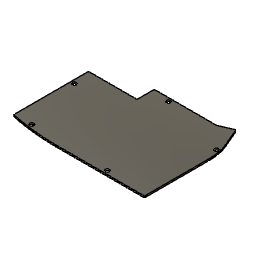
bottom plate lily58 v7 (Autodesk Fusion 360 design; units mm, degrees)
Autodesk Fusion 360 part; units mm, degrees
note: some values were not read from the file. Set by a fixed rule: which sketch regions a step uses.
sketch "bottom plate template" plane through (0, 0, 0) normal (0, 0, 1) x (1, 0, 0)
  line L0 (-42.4011, 43.5515) -> (-42.2701, 43.5244)
  line L1 (-42.5272, 43.5961) -> (-42.4011, 43.5515)
  line L2 (-42.2701, 43.5244) -> (-42.1367, 43.5153)
  line L3 (-55.1253, 50.5809) -> (-54.9545, 50.5783)
  line L4 (-64.5273, 28.4738) -> (-65.371, 25.3295)
  line L5 (-66.7867, 15.6775) -> (-66.8817, 12.4194)
  line L6 (-55.5934, 50.1095) -> (-62.3002, 34.5844)
  line L7 (-41.9037, 44.9516) -> (-41.9486, 44.9547)
  line L8 (-41.9486, 44.9547) -> (-42.014, 44.9682)
  line L9 (-42.1092, 45.0018) -> (-54.8288, 50.4967)
  line L10 (-63.502, 31.5638) -> (-64.5273, 28.4738)
  line L11 (-54.9545, 50.5783) -> (-55.1711, 50.5238)
  line L12 (-65.371, 25.3295) -> (-66.0302, 22.1414)
  line L13 (-55.1711, 50.5238) -> (-55.3484, 50.4249)
  line L14 (-55.4828, 50.2945) -> (-55.5934, 50.1095)
  line L15 (-66.0302, 22.1414) -> (-66.5026, 18.9204)
  line L16 (19.5634, 28.0336) -> (19.4331, 28.1336)
  line L17 (19.2505, 44.285) -> (19.2271, 44.463)
  line L18 (19.2711, 28.414) -> (19.2505, 28.5705)
  line L19 (19.2271, 44.463) -> (19.1628, 44.6182)
  line L20 (-66.8598, -50.3716) -> (-66.7963, -50.5251)
  line L21 (19.2505, 28.5705) -> (19.2505, 44.285)
  line L22 (66.8473, 27.4924) -> (66.7857, 27.641)
  line L23 (-62.3002, 34.5844) -> (-63.502, 31.5638)
  line L24 (19.4331, 28.1336) -> (19.3335, 28.2635)
  line L25 (25.9383, -50.737) -> (32.7303, -50.4296)
  line L26 (66.8528, -45.3702) -> (66.8694, -45.2242)
  line L27 (66.8694, -45.2242) -> (66.8694, 27.3244)
  line L28 (-42.014, 44.9682) -> (-42.1092, 45.0018)
  line L29 (-54.8288, 50.4967) -> (-55.1253, 50.5809)
  line L30 (39.5099, -49.9176) -> (46.2711, -49.2014)
  line L31 (-66.8817, 12.4194) -> (-66.8817, -50.2057)
  line L32 (-66.5666, -50.755) -> (-66.4167, -50.8171)
  line L33 (66.2436, 27.9503) -> (19.8699, 27.9503)
  line L34 (19.1392, -50.8395) -> (25.9383, -50.737)
  line L35 (19.1628, 44.6182) -> (19.0586, 44.754)
  line L36 (-66.6961, -50.6556) -> (-66.5666, -50.755)
  line L37 (-55.3484, 50.4249) -> (-55.4828, 50.2945)
  line L38 (66.8694, 27.3244) -> (66.8473, 27.4924)
  line L39 (19.0586, 44.754) -> (18.9193, 44.8609)
  line L40 (66.5601, 27.8666) -> (66.4114, 27.9282)
  line L41 (18.5904, 44.9516) -> (-41.9037, 44.9516)
  line L42 (53.0076, -48.2817) -> (59.7132, -47.1593)
  line L43 (19.8699, 27.9503) -> (19.7156, 27.9706)
  line L44 (18.7515, 44.9304) -> (18.5904, 44.9516)
  line L45 (-66.8817, -50.2057) -> (-66.8598, -50.3716)
  line L46 (18.9193, 44.8609) -> (18.7515, 44.9304)
  line L47 (-66.246, -50.8395) -> (19.1392, -50.8395)
  line L48 (19.7156, 27.9706) -> (19.5634, 28.0336)
  line L49 (-66.7963, -50.5251) -> (-66.6961, -50.6556)
  line L50 (66.7857, 27.641) -> (66.6878, 27.7686)
  line L51 (66.4114, 27.9282) -> (66.2436, 27.9503)
  line L52 (19.3335, 28.2635) -> (19.2711, 28.414)
  line L53 (66.8063, -45.5016) -> (66.8528, -45.3702)
  line L54 (66.632, -45.7171) -> (66.7315, -45.6193)
  line L55 (59.7132, -47.1593) -> (66.3751, -45.8367)
  line L56 (46.2711, -49.2014) -> (53.0076, -48.2817)
  line L57 (66.5131, -45.7902) -> (66.632, -45.7171)
  line L58 (66.7315, -45.6193) -> (66.8063, -45.5016)
  line L59 (66.6878, 27.7686) -> (66.5601, 27.8666)
  line L60 (66.3751, -45.8367) -> (66.5131, -45.7902)
  line L61 (32.7303, -50.4296) -> (39.5099, -49.9176)
  line L62 (-66.5026, 18.9204) -> (-66.7867, 15.6775)
  line L63 (-66.4167, -50.8171) -> (-66.246, -50.8395)
  circle A0 centre (1.8529, 41.4534) radius 1.5
  circle A1 centre (63.2875, 10.5583) radius 1.5
  circle A2 centre (49.4779, -45.0902) radius 1.5
  circle A3 centre (-26.7221, -47.1013) radius 1.5
  circle A4 centre (-62.68, 23.9748) radius 1.5
  circle A5 centre (-62.68, 23.9748) radius 2
  circle A6 centre (1.8529, 41.4534) radius 2
  circle A7 centre (49.4779, -45.0902) radius 2
  circle A8 centre (-26.7221, -47.1013) radius 2
  circle A9 centre (63.2875, 10.5583) radius 2
  line L64 (-41.9622, 44.8554) -> (-42.041, 44.8716)
  line L65 (-42.041, 44.8716) -> (-42.1457, 44.9087)
  line L66 (-42.1457, 44.9087) -> (-54.8625, 50.4023)
  line L67 (-54.8625, 50.4023) -> (-55.0418, 50.4532)
  line L68 (-55.0418, 50.4532) -> (-55.1339, 50.43)
  line L69 (-55.1339, 50.43) -> (-55.2883, 50.344)
  line L70 (-55.2883, 50.344) -> (-55.4037, 50.2319)
  line L71 (-55.4037, 50.2319) -> (-55.5042, 50.0638)
  line L72 (-55.5042, 50.0638) -> (-62.2079, 34.5461)
  line L73 (-62.2079, 34.5461) -> (-63.408, 31.5295)
  line L74 (-63.408, 31.5295) -> (-64.4315, 28.4451)
  line L75 (-64.4315, 28.4451) -> (-65.2737, 25.3064)
  line L76 (-65.2737, 25.3064) -> (-65.9317, 22.124)
  line L77 (-65.9317, 22.124) -> (-66.4033, 18.9088)
  line L78 (-66.4033, 18.9088) -> (-66.6869, 15.6717)
  line L79 (-66.6869, 15.6717) -> (-66.7817, 12.4179)
  line L80 (-66.7817, 12.4179) -> (-66.7817, -50.1991)
  line L81 (-66.7817, -50.1991) -> (-66.7624, -50.3455)
  line L82 (-66.7624, -50.3455) -> (-66.7089, -50.4747)
  line L83 (-66.7089, -50.4747) -> (-66.6248, -50.5843)
  line L84 (-66.6248, -50.5843) -> (-66.5162, -50.6676)
  line L85 (-66.5162, -50.6676) -> (-66.3905, -50.7197)
  line L86 (-66.3905, -50.7197) -> (-66.2395, -50.7395)
  line L87 (-66.2395, -50.7395) -> (19.1385, -50.7395)
  line L88 (19.1385, -50.7395) -> (25.9352, -50.6371)
  line L89 (25.9352, -50.6371) -> (32.7243, -50.3298)
  line L90 (32.7243, -50.3298) -> (39.5009, -49.818)
  line L91 (39.5009, -49.818) -> (46.2591, -49.1021)
  line L92 (46.2591, -49.1021) -> (52.9925, -48.1828)
  line L93 (52.9925, -48.1828) -> (59.6952, -47.0609)
  line L94 (59.6952, -47.0609) -> (66.3493, -45.7398)
  line L95 (66.3493, -45.7398) -> (66.4705, -45.6991)
  line L96 (66.4705, -45.6991) -> (66.57, -45.6379)
  line L97 (66.57, -45.6379) -> (66.6532, -45.556)
  line L98 (66.6532, -45.556) -> (66.7158, -45.4576)
  line L99 (66.7158, -45.4576) -> (66.7547, -45.3476)
  line L100 (66.7547, -45.3476) -> (66.7694, -45.2185)
  line L101 (66.7694, -45.2185) -> (66.7694, 27.3178)
  line L102 (66.7694, 27.3178) -> (66.7498, 27.4663)
  line L103 (66.7498, 27.4663) -> (66.6984, 27.5906)
  line L104 (66.6984, 27.5906) -> (66.6165, 27.6973)
  line L105 (66.6165, 27.6973) -> (66.5097, 27.7792)
  line L106 (66.5097, 27.7792) -> (66.3853, 27.8308)
  line L107 (66.3853, 27.8308) -> (66.2371, 27.8503)
  line L108 (66.2371, 27.8503) -> (19.8634, 27.8503)
  line L109 (19.8634, 27.8503) -> (19.6895, 27.8732)
  line L110 (19.6895, 27.8732) -> (19.513, 27.9463)
  line L111 (19.513, 27.9463) -> (19.3618, 28.0623)
  line L112 (19.3618, 28.0623) -> (19.2461, 28.2131)
  line L113 (19.2461, 28.2131) -> (19.1737, 28.3878)
  line L114 (19.1737, 28.3878) -> (19.1505, 28.564)
  line L115 (19.1505, 28.564) -> (19.1505, 44.2785)
  line L116 (19.1505, 44.2785) -> (19.1297, 44.4369)
  line L117 (19.1297, 44.4369) -> (19.0755, 44.5677)
  line L118 (19.0755, 44.5677) -> (18.9873, 44.6827)
  line L119 (18.9873, 44.6827) -> (18.8689, 44.7735)
  line L120 (18.8689, 44.7735) -> (18.7254, 44.833)
  line L121 (18.7254, 44.833) -> (18.5838, 44.8516)
  line L122 (18.5838, 44.8516) -> (-41.9071, 44.8516)
  line L123 (-41.9071, 44.8516) -> (-41.9622, 44.8554)
  dimension "d5" = -0.1
  dimension "d6" = 0.5
  dimension "d7" = 0.5
  dimension "d8" = 0.5
  dimension "d9" = 0.5
  dimension "d15" = 0.5
extrude "Extrude3" add sketch "bottom plate template" along normal blind 1.5 contours L64 L65 L66 L67 L68 L69 L70 L71 L72 L73 L74 L75 L76 L77 L78 L79 L80 L81 L82 L83 L84 L85 L86 L87 L88 L89 L90 L91 L92 L93 L94 L95 L96 L97 L98 L99 L100 L101 L102 L103 L104 L105 L106 L107 L108 L109 L110 L111 L112 L113 L114 L115 L116 L117 L118 L119 L120 L121 L122 L123 makes body 1
move_body "Move1" bodies 1 to x (1, 0, 0) y (0, 1, 0) z (0, 0, 1) at (85, 0, 0)
mirror "Mirror1" about plane through (0, 0, 0) normal (1, 0, 0) of bodies 1 makes body 2
delete_body "RemoveBody1" bodies 1
move_body "Move2" bodies 2 to x (1, 0, 0) y (0, 1, 0) z (0, 0, 1) at (60, 0, 0)
